Autodesk Inventor part; units mm, degrees
(part 2 of 2)
  spline S159 degree 2 poles (30.1285, -81.8356) (30.1285, -83.2435) (28.5106, -84.9231) (27.0533, -84.9231) knots 0 0 0 1 2 2 2
  spline S160 degree 2 poles (27.0533, -84.9231) (25.738, -84.9231) (24.4042, -83.4967) (24.4042, -82.1752) knots 0 0 0 1 2 2 2
  line L114 (24.4042, -82.1752) -> (24.4042, -81.5268)
  line L115 (24.4042, -81.5268) -> (28.3377, -81.5268)
  spline S161 degree 2 poles (28.3377, -81.5268) (28.313, -81.1255) (28.0228, -80.5944) (27.7881, -80.4339) knots 0 0 0 1 2 2 2
  spline S162 degree 2 poles (27.7881, -80.4339) (27.5597, -80.2733) (26.9422, -80.1374) (26.5778, -80.1374) knots 0 0 0 1 2 2 2
  spline S163 degree 2 poles (26.5778, -80.1374) (26.2691, -80.1374) (25.6639, -80.2733) (25.4108, -80.3906) knots 0 0 0 1 2 2 2
  spline S164 degree 2 poles (25.4108, -80.3906) (25.1885, -80.4833) (24.8179, -80.7117) (24.7006, -80.7982) knots 0 0 0 1 2 2 2
  line L116 (24.7006, -80.7982) -> (24.5092, -80.7982)
  line L117 (24.5092, -80.7982) -> (24.5092, -79.3162)
  spline S165 degree 2 poles (24.5092, -79.3162) (24.7315, -79.2297) (25.0896, -79.0815) (25.4108, -79.0074) knots 0 0 0 1 2 2 2
  spline S166 degree 2 poles (25.4108, -79.0074) (25.701, -78.9271) (26.3185, -78.8407) (26.7631, -78.8407) knots 0 0 0 1 2 2 2
  spline S167 degree 2 poles (26.1703, -82.6075) (26.1826, -83.1756) (26.6828, -83.7745) (27.1953, -83.7745) knots 0 0 0 1 2 2 2
  spline S168 degree 2 poles (27.1953, -83.7745) (27.7202, -83.7745) (28.313, -83.1447) (28.3439, -82.6075) knots 0 0 0 1 2 2 2
  line L118 (28.3439, -82.6075) -> (26.1703, -82.6075)
  line L119 (55.5233, -74.0317) -> (58.1416, -66.4117)
  line L120 (58.1416, -66.4117) -> (60.1361, -66.4117)
  line L121 (60.1361, -66.4117) -> (62.7543, -74.0317)
  line L122 (62.7543, -74.0317) -> (60.7721, -74.0317)
  line L123 (60.7721, -74.0317) -> (59.111, -68.8632)
  line L124 (59.111, -68.8632) -> (57.4561, -74.0317)
  line L125 (57.4561, -74.0317) -> (55.5233, -74.0317)
  spline S169 degree 2 poles (49.1692, -70.2217) (49.1692, -69.2337) (49.4841, -67.7517) (49.8361, -67.2515) knots 0 0 0 1 2 2 2
  spline S170 degree 2 poles (49.8361, -67.2515) (50.1819, -66.7575) (51.2996, -66.2512) (52.1024, -66.2512) knots 0 0 0 1 2 2 2
  spline S171 degree 2 poles (52.1024, -66.2512) (52.9113, -66.2512) (54.0228, -66.7575) (54.3748, -67.2639) knots 0 0 0 1 2 2 2
  spline S172 degree 2 poles (54.3748, -67.2639) (54.7268, -67.764) (55.0417, -69.2337) (55.0417, -70.2217) knots 0 0 0 1 2 2 2
  spline S173 degree 2 poles (55.0417, -70.2217) (55.0417, -71.2344) (54.7268, -72.667) (54.3686, -73.1857) knots 0 0 0 1 2 2 2
  spline S174 degree 2 poles (54.3686, -73.1857) (54.0105, -73.6921) (52.8804, -74.1861) (52.1024, -74.1861) knots 0 0 0 1 2 2 2
  spline S175 degree 2 poles (52.1024, -74.1861) (51.2811, -74.1861) (50.1819, -73.6674) (49.8299, -73.1549) knots 0 0 0 1 2 2 2
  spline S176 degree 2 poles (49.8299, -73.1549) (49.4841, -72.6547) (49.1692, -71.1788) (49.1692, -70.2217) knots 0 0 0 1 2 2 2
  spline S177 degree 2 poles (51.0897, -70.2217) (51.0897, -71.6358) (51.5528, -72.7782) (52.1024, -72.7782) knots 0 0 0 1 2 2 2
  spline S178 degree 2 poles (52.1024, -72.7782) (52.6519, -72.7782) (53.1212, -71.6358) (53.1212, -70.2155) knots 0 0 0 1 2 2 2
  spline S179 degree 2 poles (53.1212, -70.2155) (53.1212, -68.82) (52.6519, -67.6591) (52.1024, -67.6591) knots 0 0 0 1 2 2 2
  spline S180 degree 2 poles (52.1024, -67.6591) (51.559, -67.6591) (51.0897, -68.82) (51.0897, -70.2217) knots 0 0 0 1 2 2 2
  spline S181 degree 2 poles (42.5866, -68.7212) (42.5866, -68.1592) (43.0004, -67.2392) (43.4017, -66.9181) knots 0 0 0 1 2 2 2
  spline S182 degree 2 poles (43.4017, -66.9181) (43.8031, -66.597) (44.8961, -66.2512) (45.6803, -66.2512) knots 0 0 0 1 2 2 2
  spline S183 degree 2 poles (45.6803, -66.2512) (46.5695, -66.2512) (47.8416, -66.5476) (48.243, -66.7328) knots 0 0 0 1 2 2 2
  line L126 (48.243, -66.7328) -> (48.243, -68.3877)
  line L127 (48.243, -68.3877) -> (48.0577, -68.3877)
  spline S184 degree 2 poles (48.0577, -68.3877) (47.6378, -68.1222) (46.5078, -67.727) (46.0385, -67.727) knots 0 0 0 1 2 2 2
  spline S185 degree 2 poles (46.0385, -67.727) (45.7606, -67.727) (45.1122, -67.8258) (44.8899, -67.9863) knots 0 0 0 1 2 2 2
  spline S186 degree 2 poles (44.8899, -67.9863) (44.717, -68.116) (44.5071, -68.4927) (44.5071, -68.8323) knots 0 0 0 1 2 2 2
  spline S187 degree 2 poles (44.5071, -68.8323) (44.5071, -69.172) (44.8035, -69.5363) (45.0505, -69.6227) knots 0 0 0 1 2 2 2
  spline S188 degree 2 poles (45.0505, -69.6227) (45.2975, -69.7092) (45.9829, -69.7277) (46.2484, -69.7277) knots 0 0 0 1 2 2 2
  line L128 (46.2484, -69.7277) -> (46.5757, -69.7277)
  line L129 (46.5757, -69.7277) -> (46.5757, -71.0677)
  line L130 (46.5757, -71.0677) -> (46.2731, -71.0677)
  spline S189 degree 2 poles (46.2731, -71.0677) (45.9273, -71.0677) (45.3407, -71.1294) (45.1369, -71.2221) knots 0 0 0 1 2 2 2
  spline S190 degree 2 poles (45.1369, -71.2221) (44.9331, -71.3209) (44.7047, -71.6667) (44.7047, -71.9631) knots 0 0 0 1 2 2 2
  spline S191 degree 2 poles (44.7047, -71.9631) (44.7047, -72.1977) (44.9208, -72.4879) (45.0752, -72.5682) knots 0 0 0 1 2 2 2
  spline S192 degree 2 poles (45.0752, -72.5682) (45.2604, -72.6608) (45.7544, -72.7226) (45.9273, -72.7226) knots 0 0 0 1 2 2 2
  spline S193 degree 2 poles (45.9273, -72.7226) (46.2052, -72.7226) (46.7918, -72.5929) (47.0635, -72.4879) knots 0 0 0 1 2 2 2
  spline S194 degree 2 poles (47.0635, -72.4879) (47.2797, -72.4077) (47.749, -72.1483) (47.8601, -72.0804) knots 0 0 0 1 2 2 2
  line L131 (47.8601, -72.0804) -> (48.0207, -72.0804)
  line L132 (48.0207, -72.0804) -> (48.0207, -73.7106)
  spline S195 degree 2 poles (48.0207, -73.7106) (47.6255, -73.8773) (46.2917, -74.1923) (45.5939, -74.1923) knots 0 0 0 1 2 2 2
  spline S196 degree 2 poles (45.5939, -74.1923) (44.9146, -74.1923) (43.9143, -73.9576) (43.5623, -73.7291) knots 0 0 0 1 2 2 2
  spline S197 degree 2 poles (43.5623, -73.7291) (43.1733, -73.4883) (42.7842, -72.7473) (42.7842, -72.2842) knots 0 0 0 1 2 2 2
  spline S198 degree 2 poles (42.7842, -72.2842) (42.7842, -71.6296) (43.5376, -70.654) (44.1551, -70.5119) knots 0 0 0 1 2 2 2
  line L133 (44.1551, -70.5119) -> (44.1551, -70.4378)
  spline S199 degree 2 poles (44.1551, -70.4378) (43.8834, -70.4008) (43.3647, -70.2032) (43.1177, -69.9809) knots 0 0 0 1 2 2 2
  spline S200 degree 2 poles (43.1177, -69.9809) (42.8892, -69.7833) (42.5866, -69.1534) (42.5866, -68.7212) knots 0 0 0 1 2 2 2
  point P0 (52.4636, -6.35)
  constraints: 2 end point, 2 midpoint, 1 horizontal
extrude "Name and Version Number" cut sketch "Sketch15" against normal blind 3.175
equation "\"d14\" = gapBetweenParts"
equation "\"d16\" = gapBetweenParts"
equation "\"d18\" = gapBetweenParts"
equation "\"d20\" = gapBetweenParts"
equation "\"d21\" = gapBetweenParts"
equation "\"gapBetweenParts\" = 6.35"
body "Solid3"
